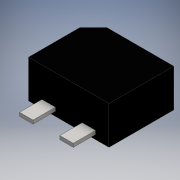
# Autodesk Inventor part: QRE1113
Saved by Autodesk Inventor 2016 (Build 200138000, 138)
## iProperties
Created: 2016-01-30
Part Number: QRE1113
Material: Generic
Document SubType Name: Modeling
Designer: jferner
Density: 1 g/cm^3
Appearance: Default
QRE1113_z: 1.700 mm
QRE1113_y: 3.600 mm
QRE1113_x: 2.900 mm
Author: jferner
Autodesk Inventor part; units mm, degrees
ref_plane "YZ Plane" through (0, 0, 0) normal (1, 0, 0) x (0, 1, 0)
ref_plane "XZ Plane" through (0, 0, 0) normal (0, 1, 0) x (-1, 0, 0)
ref_plane "XY Plane" through (0, 0, 0) normal (0, 0, 1) x (1, 0, 0)
sketch "Sketch1" plane through (0, 0, 0) normal (0, 0, 1) x (1, 0, 0)
  line L0 (0, 0) -> (3.6, 0)
  line L1 (3.6, 0) -> (3.6, 2.9)
  line L2 (3.6, 2.9) -> (0.6, 2.9)
  line L3 (0, 2.3) -> (0, 0)
  line L4 (0.6, 2.9) -> (0, 2.3)
  dimension "QRE1113_x" = 2.9
  dimension "d2" = 135
  dimension "d3" = 3
  dimension "QRE1113_y" = 3.6
  constraints: 10 end point, 2 parallel, 1 horizontal, 1 perpendicular
  measures "QRE1113_x" distance of L0.end L1.end
  measures "d2" angle of L2 L4
  measures "d3" distance of L2.end L1.end
  measures "QRE1113_y" distance between parallel lines of L1 L3
extrude "Extrusion1" add sketch "Sketch1" along normal blind 1.7
sketch "Sketch2" plane through (0, 0, 0) normal (0, -1, 0) x (1, 0, 0)
  line L0 (0.6, 0.36) -> (1.2, 0.36)
  line L1 (1.2, 0.36) -> (1.2, 0.2)
  line L2 (1.2, 0.2) -> (0.6, 0.2)
  line L3 (0.6, 0.2) -> (0.6, 0.36)
  line L4 (2.4, 0.36) -> (3, 0.36)
  line L5 (3, 0.36) -> (3, 0.2)
  line L6 (3, 0.2) -> (2.4, 0.2)
  line L7 (2.4, 0.2) -> (2.4, 0.36)
  line L8 (0, 0) -> (0, 1.7) projected
  line L9 (3.6, 0) -> (3.6, 1.7) projected
  line L10 (0, 0) -> (3.6, 0) projected
  dimension "d7" = 0.6
  dimension "d8" = 0.6
  dimension "d9" = 0.6
  dimension "d10" = 0.2
  dimension "d11" = 0.16
  constraints: 16 end point, 4 parallel, 2 horizontal, 2 perpendicular, 2 point on line, 1 collinear
  measures "d7" distance of L0.start L0.end
  measures "d8" distance between parallel lines of L3 L8
  measures "d9" distance between parallel lines of L9 L5
  measures "d10" distance between parallel lines of L10 L2
  measures "d11" distance of L2.end L0.start
extrude "Extrusion2" add sketch "Sketch2" along normal blind 1
body "Solid1"
